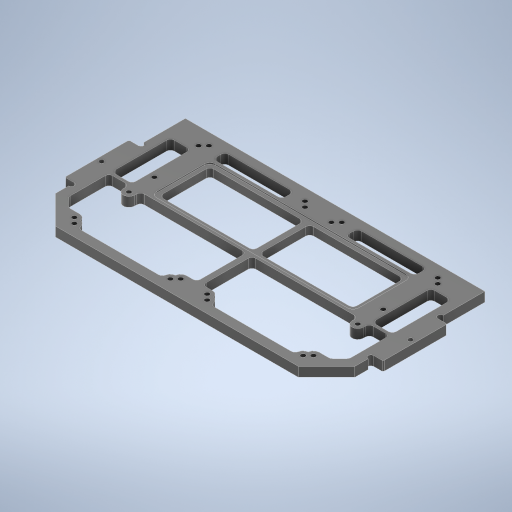
# Autodesk Inventor part: TorsoElectronicBoxBoardMountFrame
Saved by Autodesk Inventor 2024.2 (Build 282272000, 272)
## iProperties
Created: 2024-01-11
Part Number: TorsoElectronicBoxBoardMountFrame
Material: Acetal Resin, Black
Document SubType Name: Modeling
Designer: Masato Kubotera
Density: 1.425 g/cm^3
Appearance: Smooth - Black
Vendor: meviy
Mass: 32.4012 g
Surface Area: 177.402 cm^2
Volume: 22.7377 cm^3
Author: Masato Kubotera
Autodesk Inventor part; units mm, degrees
ref_plane "YZ Plane" through (0, 0, 0) normal (1, 0, 0) x (0, 1, 0)
ref_plane "XZ Plane" through (0, 0, 0) normal (0, 1, 0) x (-1, 0, 0)
ref_plane "XY Plane" through (0, 0, 0) normal (0, 0, 1) x (1, 0, 0)
sketch "Sketch1" plane through (0, 0, 0) normal (0, 0, 1) x (1, 0, 0)
  line L0 (-42, -79.5) -> (42, -79.5)
  line L1 (42, -79.5) -> (42, 79.5)
  line L2 (42, 79.5) -> (-42, 79.5) construction
  line L3 (-42, 79.5) -> (-42, -79.5)
  line L4 (-42, -79.5) -> (42, 79.5) construction
  line L5 (42, -79.5) -> (-42, 79.5) construction
  line L6 (-42, 0) -> (42, 0)
  line L7 (-17, 84.5) -> (17, 84.5)
  line L8 (17, 84.5) -> (17, 79.5)
  line L9 (-17, 84.5) -> (-17, 79.5)
  arc A0 (-20, 79.5) -> (-17, 79.5) centre (-18.5, 79.5) ccw
  line L10 (17, 84.5) -> (17, 79.5)
  arc A1 (17, 79.5) -> (20, 79.5) centre (18.5, 79.5) ccw
  line L11 (0, 79.5) -> (0, 84.5) construction
  line L12 (0, -70) -> (0, 70) construction
  line L13 (-33, 7) -> (33, 7) construction
  line L14 (33, 7) -> (33, 63.5) construction
  line L15 (33, 63.5) -> (-33, 63.5) construction
  line L16 (-33, 63.5) -> (-33, 7) construction
  line L17 (-33, 7) -> (33, 63.5) construction
  line L18 (33, 7) -> (-33, 63.5) construction
  line L19 (-40, 2.75) -> (40, 2.75) construction
  line L20 (40, 2.75) -> (40, 67.75) construction
  line L21 (40, 67.75) -> (-40, 67.75) construction
  line L22 (-40, 67.75) -> (-40, 2.75) construction
  line L23 (-40, 2.75) -> (40, 67.75) construction
  line L24 (40, 2.75) -> (-40, 67.75) construction
  line L25 (-40, 35.25) -> (40, 35.25) construction
  line L26 (5.6, 74.5) -> (24.1005, 74.5)
  arc A2 (35.3, 12.7161) -> (37, 14.6934) centre (35, 14.6934) ccw
  arc A3 (28, 1.5) -> (30, 3.5) centre (28, 3.5) ccw
  line L27 (-42, 79.5) -> (-20, 79.5)
  line L28 (20, 79.5) -> (42, 79.5)
  line L29 (-26, -53.5) -> (-1, -53.5) construction
  line L30 (2, -50.5) -> (2, 50.5) construction
  line L31 (-1, 53.5) -> (-26, 53.5) construction
  line L32 (-29, 50.5) -> (-29, -50.5) construction
  arc A4 (-26, 53.5) -> (-29, 50.5) centre (-26, 50.5) ccw construction
  arc A5 (2, 50.5) -> (-1, 53.5) centre (-1, 50.5) ccw construction
  arc A6 (-29, -50.5) -> (-26, -53.5) centre (-26, -50.5) ccw construction
  arc A7 (-1, -53.5) -> (2, -50.5) centre (-1, -50.5) ccw construction
  line L33 (-29, 0) -> (2, 0) construction
  circle A8 centre (-33, 7) radius 3 construction
  line L34 (-13.5, 53.5) -> (-13.5, -53.5) construction
  line L35 (5.6, 1.5) -> (28, 1.5)
  arc A9 (5.6, 74.5) -> (3.6, 72.5) centre (5.6, 72.5) ccw
  line L36 (-25, 1.5) -> (-2, 1.5)
  line L37 (0, 3.5) -> (0, 49.5)
  line L38 (-2, 51.5) -> (-25, 51.5)
  line L39 (-27, 49.5) -> (-27, 3.5)
  arc A10 (-27, 3.5) -> (-25, 1.5) centre (-25, 3.5) ccw
  arc A11 (-2, 1.5) -> (0, 3.5) centre (-2, 3.5) ccw
  arc A12 (0, 49.5) -> (-2, 51.5) centre (-2, 49.5) ccw
  arc A13 (-25, 51.5) -> (-27, 49.5) centre (-25, 49.5) ccw
  arc A14 (32.7596, 60.5096) -> (35.3, 57.7839) centre (35.75, 60.75) ccw
  arc A15 (37, 55.8066) -> (35.3, 57.7839) centre (35, 55.8066) ccw
  line L40 (37, 55.8066) -> (37, 14.6934)
  arc A16 (35.3, 12.7161) -> (32.7596, 9.9904) centre (35.75, 9.75) ccw
  line L41 (-29.1, 0) -> (-29.1, 50.6)
  line L42 (-26.1, 53.6) -> (-0.9, 53.6)
  line L43 (2.1, 50.6) -> (2.1, 0)
  arc A17 (2.1, 50.6) -> (-0.9, 53.6) centre (-0.9, 50.6) ccw
  arc A18 (-26.1, 53.6) -> (-29.1, 50.6) centre (-26.1, 50.6) ccw
  arc A19 (3.6, 3.5) -> (5.6, 1.5) centre (5.6, 3.5) ccw
  line L44 (-27.1, 63.75) -> (0.1, 63.75)
  line L45 (2.1, 65.75) -> (2.1, 72.5)
  line L46 (0.1, 74.5) -> (-27.1, 74.5)
  line L47 (-29.1, 72.5) -> (-29.1, 65.75)
  line L48 (-35, 16.9) -> (-32.6, 16.9)
  line L49 (-30.6, 18.9) -> (-30.6, 51.6)
  line L50 (-32.6, 53.6) -> (-35, 53.6)
  line L51 (-37, 51.6) -> (-37, 18.9)
  circle A20 centre (-35.75, 9.75) radius 3 construction
  circle A21 centre (-35.75, 60.75) radius 3 construction
  arc A22 (-29.1, 65.75) -> (-27.1, 63.75) centre (-27.1, 65.75) ccw
  arc A23 (0.1, 63.75) -> (2.1, 65.75) centre (0.1, 65.75) ccw
  arc A24 (2.1, 72.5) -> (0.1, 74.5) centre (0.1, 72.5) ccw
  arc A25 (-27.1, 74.5) -> (-29.1, 72.5) centre (-27.1, 72.5) ccw
  arc A26 (-30.6, 51.6) -> (-32.6, 53.6) centre (-32.6, 51.6) ccw
  arc A27 (-35, 53.6) -> (-37, 51.6) centre (-35, 51.6) ccw
  arc A28 (-37, 18.9) -> (-35, 16.9) centre (-35, 18.9) ccw
  arc A29 (-32.6, 16.9) -> (-30.6, 18.9) centre (-32.6, 18.9) ccw
  line L52 (27, 79.5) -> (42, 64.5)
  line L53 (29.4142, 70.0147) -> (25.5147, 73.9142)
  arc A30 (30, 68.6005) -> (29.4142, 70.0147) centre (28, 68.6005) ccw
  arc A31 (25.5147, 73.9142) -> (24.1005, 74.5) centre (24.1005, 72.5) ccw
  circle A32 centre (33, 7) radius 3 construction
  line L54 (6.75, 9.75) -> (35.75, 9.75) construction
  line L55 (35.75, 9.75) -> (35.75, 60.75) construction
  line L56 (35.75, 60.75) -> (6.75, 60.75) construction
  line L57 (6.75, 60.75) -> (6.75, 9.75) construction
  line L58 (6.75, 9.75) -> (35.75, 60.75) construction
  line L59 (35.75, 9.75) -> (6.75, 60.75) construction
  arc A33 (32.7596, 9.9904) -> (30, 7) centre (33, 7) ccw
  line L60 (30, 3.5) -> (30, 7)
  arc A34 (32.7596, 60.5096) -> (35.3, 57.7839) centre (35.75, 60.75) ccw
  arc A35 (30, 63.5) -> (32.7596, 60.5096) centre (33, 63.5) ccw
  line L61 (30, 68.6005) -> (30, 63.5)
  arc A36 (6.75, 57.75) -> (6.75, 63.75) centre (6.75, 60.75) ccw
  line L62 (6.75, 57.75) -> (5.6, 57.75)
  line L63 (6.75, 63.75) -> (5.6, 63.75)
  line L64 (3.6, 3.5) -> (3.6, 55.75)
  line L65 (3.6, 65.75) -> (3.6, 72.5)
  arc A37 (5.6, 57.75) -> (3.6, 55.75) centre (5.6, 55.75) ccw
  arc A38 (3.6, 65.75) -> (5.6, 63.75) centre (5.6, 65.75) ccw
  point P0 (0, 0)
  point P1 (0, 35.25)
  point P2 (0, 82)
  point P3 (-29, -53.5)
  point P4 (2, -53.5)
  point P5 (-29.1, 63.75)
  point P6 (2.1, 74.5)
  point P7 (2.1, 63.75)
  point P8 (-29.1, 74.5)
  point P9 (-37, 16.9)
  point P10 (-30.6, 53.6)
  point P11 (-30.6, 16.9)
  point P12 (-37, 53.6)
  point P13 (21.25, 35.25)
  point P14 (-6.75, 60.75)
  point P15 (3.6, 57.75)
  point P16 (3.6, 63.75)
  dimension "d1" = 159
  dimension "d2" = 1.5
  dimension "d3" = 5
  dimension "d36" = 25
  dimension "d42" = 56.5
  dimension "d43" = 66
  dimension "d44" = 80
  dimension "d45" = 65
  dimension "d67" = 5
  dimension "d70" = 42
  dimension "d71" = 84
  dimension "d73" = 25
  dimension "d75" = 14
  dimension "d95" = 3
  dimension "d97" = 31
  dimension "d100" = 107
  dimension "d102" = 6
  dimension "d103" = 1
  dimension "d108" = 3
  dimension "d113" = 2
  dimension "d114" = 2
  dimension "d115" = 2
  dimension "d116" = 5
  dimension "d118" = 6
  dimension "d122" = 2
  dimension "d123" = 0.1
  dimension "d124" = 0.1
  dimension "d147" = 15
  dimension "d148" = 45
  dimension "d150" = 5
  dimension "d151" = 51
  dimension "d152" = 4.25
  dimension "d153" = 29
  dimension "d154" = 1.5
  constraints: 132 end point, 70 point on circle, 57 tangent, 38 centre point, 34 point on line, 27 equal radius, 20 midpoint, 15 horizontal, 15 parallel, 13 coincident, 11 symmetric about line, 11 vertical, 9 collinear, 7 perpendicular, 15 other
  measures "d1" distance of L1.end L0.end
  measures "d2" radius of A0
  measures "d3" distance of L7.start L9.end
  measures "d36" distance between parallel lines of L8 L1
  measures "d42" distance of L15.end L13.start
  measures "d43" distance of L14.end L15.end
  measures "d44" distance of L21.end L20.end
  measures "d45" distance of L19.end L20.end
  measures "d67" distance between parallel lines of L2 L26
  measures "d70" distance between parallel lines of L1 L12
  measures "d71" distance between parallel lines of L1 L3
  measures "d73" distance between parallel lines of L9 L3
  measures "d75" diameter of point (-33, 7) L6
  measures "d95" radius of A4
  measures "d97" distance of point (-29, -53.5) point (2, -53.5)
  measures "d100" distance between parallel lines of L31 L29
  measures "d102" diameter of A8
  measures "d103" distance edge to line of A8 L32
  measures "d108" diameter of L35 L6
  measures "d113" radius of A10
  measures "d114" distance between parallel lines of L30 L37
  measures "d115" distance between parallel lines of L31 L38
  measures "d116" distance between parallel lines of L1 L40
  measures "d118" diameter of A16
  measures "d122" radius of A3
  measures "d123" distance between parallel lines of L43 L30
  measures "d124" distance between parallel lines of L42 L31
  measures "d147" distance of L1.end L52.end
  measures "d148" angle of L1 L52
  measures "d150" distance between parallel lines of L52 L53
  measures "d151" distance of A14.centre point (35.75, 9.75)
  measures "d152" distance from line of L20 point (35.75, 9.75)
  measures "d153" distance of L55.end L56.end
  measures "d154" distance between parallel lines of L64 L43
extrude "Extrusion1" add sketch "Sketch1" against normal blind 5 contours L3 L27 A0 L9 L7 L8 A1 L28 L52 L1 L6 L43 A17 L42 A18 L41 | L41 A18 L42 A17 L43 L6
extrude "Extrusion2" cut sketch "Sketch1" against normal blind 0.7 contours L41 A18 L42 A17 L43 L6
chamfer "C0.5" distance 0.5 angle 45 2 edges at (17, 84.5, -2.5) (-17, 84.5, -2.5)
hole "M3" at (-33, 7, 0) at (-33, 63.5, 0) at (33, 7, 0) at (33, 63.5, 0) at (35.75, 9.75, 0) at (35.75, 60.75, 0) at (-35.75, 9.75, 0) at (-35.75, 60.75, 0) at (6.75, 60.75, 0) at (-6.75, 60.75, 0) direction (0, 0, -1) diameter 2.459 end through all thread size "M3x0.5" class "6H" standard "ANSI Metric M Profile"
hole "Phi2.5" at (0, 82, 0) direction (0, 0, -1) diameter 2.5 end through all
mirror "Mirror1" about plane through (0, 0, 0) normal (0, 1, 0)
ref_plane "Work Plane1" through (-13.5, 53.5, 0) normal (-1, 0, 0) x (0, 0, 1)
body "Solid1"
